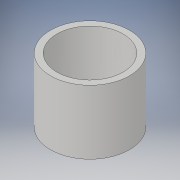
# Autodesk Inventor part: cargotrunk
Saved by Autodesk Inventor 2018 (Build 220112000, 112)
## iProperties
Created: 2018-04-21
Part Number: cargotrunk
Material: Generic
Document SubType Name: Modeling
Designer: atbin
Density: 0.231958 g/cm^3
Appearance: Default
Mass: 2.22988e+06 g
Surface Area: 704973 cm^2
Volume: 9.61327e+06 cm^3
Author: atbin
Autodesk Inventor part; units mm, degrees
ref_plane "YZ Plane" through (0, 0, 0) normal (1, 0, 0) x (0, 1, 0)
ref_plane "XZ Plane" through (0, 0, 0) normal (0, 1, 0) x (-1, 0, 0)
ref_plane "XY Plane" through (0, 0, 0) normal (0, 0, 1) x (1, 0, 0)
sketch "Sketch1" plane through (0, 0, 0) normal (0, 0, 1) x (1, 0, 0)
  line L0 (-1850, 3000) -> (-1550, 3000)
  line L1 (-1550, 3000) -> (-1550, 0)
  line L2 (-1550, 0) -> (-1850, 0)
  line L3 (-1850, 0) -> (-1850, 3000)
  line L4 (0, 3600) -> (0, -600) projected
  line L5 (-2220, 0) -> (370, 0) projected
  line L6 (0, -600) -> (0, 3600) projected
  point P0 (0, 0)
  dimension "d0" = 1550
  dimension "d1" = 1850
  dimension "d2" = 0
  dimension "d3" = 3000
  constraints: 8 end point, 2 parallel, 1 horizontal, 1 perpendicular
  measures "d0" distance between parallel lines of L4 L1
  measures "d1" distance between parallel lines of L4 L3
  measures "d2" distance between parallel lines of L5 L2
  measures "d3" distance between parallel lines of L0 L2
revolve "Revolution1" add sketch "Sketch1" angle 360 about axis through (0, -10, 0) along (0, 1, 0)
body "Solid1"
